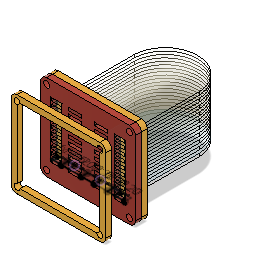
number_base_space_50mm_3mm_2mm v16 (Autodesk Fusion 360 design; units mm, degrees)
Autodesk Fusion 360 part; units mm, degrees
note: some values were not read from the file. Set by a fixed rule: which face or edge a step refers to.
(part 1 of 2)
sketch "Skizze1" plane through (0, 0, 0) normal (0, 1, 0) x (1, 0, 0)
  line L0 (0, 0) -> (43.75, 0)
  line L1 (43.75, 0) -> (43.75, -70)
  line L2 (43.75, -70) -> (0, -70)
  line L3 (0, -70) -> (0, 0)
  line L4 (36.1216, -93.0117) -> (36.1102, -92.9933) construction
  arc A0 (43.75, -23.3333) -> (0, -23.3333) centre (21.875, -21.9206) ccw
  line L5 (0, -70) -> (4, -70)
  line L6 (4, -70) -> (4, -74)
  line L7 (4, -74) -> (0, -74)
  line L8 (0, -74) -> (0, -70)
  line L9 (39.75, -70) -> (43.75, -70)
  line L10 (43.75, -70) -> (43.75, -74)
  line L11 (43.75, -74) -> (39.75, -74)
  line L12 (39.75, -74) -> (39.75, -70)
  line L13 (8.75, -70) -> (17.5, -70)
  line L14 (17.5, -70) -> (17.5, -74)
  line L15 (17.5, -74) -> (8.75, -74)
  line L16 (8.75, -74) -> (8.75, -70)
  line L17 (26.25, -70) -> (35, -70)
  line L18 (35, -70) -> (35, -74)
  line L19 (35, -74) -> (26.25, -74)
  line L20 (26.25, -74) -> (26.25, -70)
  line L21 (4, -70) -> (2.5, -70)
  line L22 (2.5029, -74) -> (4, -74)
  line L23 (4, -74) -> (4, -70)
  line L24 (39.75, -70) -> (41.25, -70)
  line L25 (39.75, -55) -> (39.75, -70)
  line L26 (43.75, -74) -> (46.75, -74)
  line L27 (46.75, -74) -> (46.75, -70)
  line L28 (46.75, -70) -> (43.75, -70)
  line L29 (43.75, -70) -> (43.75, -74)
  line L30 (0, -70) -> (-3, -70)
  line L31 (-3, -70) -> (-3, -74)
  line L32 (-3, -74) -> (0, -74)
  line L33 (0, -74) -> (0, -70)
  line L34 (-3, -70) -> (34.25, -70)
  line L35 (-3, -69.5) -> (-3, -70)
  line L36 (4, -70) -> (26.25, -70)
  line L37 (26.25, -70) -> (26.25, -74)
  line L38 (4, -74) -> (4, -70)
  line L39 (39.75, -70) -> (17.5, -70)
  line L40 (17.5, -70) -> (17.5, -74)
  line L41 (39.75, -74) -> (39.75, -70)
  point P0 (21.875, -70)
  dimension "d1" = 43.75
  dimension "d2" = 70
  dimension "d15" = 23.3333
  dimension "d16" = 23.3333
  dimension "d21" = 4
  dimension "d22" = 4
  dimension "d23" = 4
  dimension "d24" = 4
  dimension "d25" = 8.75
  dimension "d26" = 4
  dimension "d27" = 8.75
  dimension "d28" = 8.75
  dimension "d29" = 4
  dimension "d30" = 8.75
  dimension "d31" = 4
  dimension "d32" = 1.5
  dimension "d34" = 1.5
  dimension "d35" = 3
  dimension "d36" = 3
  dimension "d37" = 4
  dimension "d38" = 4
  dimension "d153" = 0.5
  constraint horizontal L0
  constraint vertical L1
  constraint horizontal L2
  constraint vertical L3
  constraint coincident L0.start L3.end
  constraint coincident L4 P0
  constraint midpoint L2 P0
  constraint coincident L3 A0.end
  constraint coincident L1 A0.start
  constraint tangent L0 A0
  constraint horizontal L5
  constraint vertical L6
  constraint horizontal L7
  constraint vertical L8
  constraint horizontal L9
  constraint vertical L10
  constraint horizontal L11
  constraint vertical L12
  constraint coincident L2 L9.start
  constraint coincident L1.end L10
  constraint horizontal L13
  constraint vertical L14
  constraint horizontal L15
  constraint vertical L16
  constraint coincident L2 L13.start
  constraint horizontal L17
  constraint vertical L18
  constraint horizontal L19
  constraint vertical L20
  constraint coincident L2 L17.start
  constraint horizontal L21
  constraint horizontal L22
  constraint vertical L23
  constraint horizontal L24
  constraint vertical L25
  constraint horizontal L26
  constraint vertical L27
  constraint horizontal L28
  constraint vertical L29
  constraint horizontal L30
  constraint vertical L31
  constraint horizontal L32
  constraint vertical L33
  constraint horizontal L34
  constraint vertical L35
  constraint horizontal L36
  constraint vertical L37
  constraint vertical L38
  constraint horizontal L39
  constraint vertical L40
  constraint vertical L41
  measures "d1" distance of L0.start L0.end
  measures "d2" distance of L0.start L2.end
  measures "d15" distance of L0.start A0.end
  measures "d16" distance of L0.end A0.start
  measures "d21" distance of L6.end L7.end
  measures "d22" distance of L10.end L11.end
  measures "d23" distance of L9.start L11.end
  measures "d24" distance of L5.end L6.end
  measures "d25" distance of L13.start L13.end
  measures "d26" distance of L13.start L15.end
  measures "d27" distance of L8 L16
  measures "d28" distance of L17.start L17.end
  measures "d29" distance of L17.start L19.end
  measures "d30" distance of L10 L18
  measures "d31" distance of L21.end L22.start
  measures "d32" distance of L5.end L21.end
  measures "d34" distance of L9.start L24.end
  measures "d35" distance of L10.end L26.end
  measures "d36" distance of L2.end L30.end
  measures "d37" distance of L26.end L27.end
  measures "d38" distance of L30.end L31.end
  measures "d153" distance of L30.end L35.start
extrude "Extrusion1" add sketch "Skizze1" along normal blind 2 contours L1 L2 L3 A0 L5 L9 L13 L17 L21 L24 L34 L36 L39 | L2 L5 L6 L7 L8 L21 L22 L23 L33 L34 L38 | L8 L30 L31 L32 L33 L34 | L2 L9 L10 L11 L12 L24 L29 L41 | L10 L26 L27 L28 L29 | L2 L13 L14 L15 L16 L34 L36 L40 | L2 L17 L18 L19 L20 L34 L37 L39 makes body 1
sketch "Skizze2" plane through (0, 0, 70) normal (0, 0, -1) x (-1, 0, 0)
  line L0 (0, 0) -> (3, 0)
  line L1 (3, 0) -> (3, 2)
  line L2 (3, 2) -> (0, 2)
  line L3 (0, 2) -> (0, 0)
  line L4 (0.1, -0.01) -> (-43.85, -0.01)
  line L5 (-43.85, -0.01) -> (-43.85, 38.01)
  line L6 (-43.85, 38.01) -> (0.1, 38.01)
  line L7 (0.1, 38.01) -> (0.1, -0.01)
  line L8 (0, 0) -> (-43.75, 0)
  line L9 (-43.75, 0) -> (-43.75, 2)
  line L10 (10.1, -10.01) -> (-53.85, -10.01)
  line L11 (-53.85, -10.01) -> (-53.85, 48.01)
  line L12 (-53.85, 48.01) -> (10.1, 48.01)
  line L13 (10.1, 48.01) -> (10.1, -10.01)
  circle A0 centre (-49.85, -6.01) radius 4
  circle A1 centre (6.1, 44.01) radius 4
  circle A2 centre (-49.85, 44.01) radius 4
  circle A3 centre (6.1, -6.01) radius 4
  circle A4 centre (6.1, -6.01) radius 2
  circle A5 centre (-49.85, -6.01) radius 2
  circle A6 centre (-49.85, 44.01) radius 2
  circle A7 centre (6.1, 44.01) radius 2
  line L14 (-80, 31) -> (-59, 31)
  line L15 (-59, 31) -> (-59, 29)
  line L16 (-59, 29) -> (-80, 29)
  line L17 (-80, 29) -> (-80, 31)
  line L18 (-100.8189, 25.8246) -> (-75.8188, 25.8008) construction
  line L19 (-75.8188, 25.8008) -> (-75.8107, 34.2225) construction
  line L20 (-75.8107, 34.2225) -> (-100.8108, 34.2463) construction
  line L21 (-100.8108, 34.2463) -> (-100.8189, 25.8246) construction
  line L22 (-81, 19) -> (-60, 19)
  line L23 (-60, 19) -> (-60, 15)
  line L24 (-60, 15) -> (-81, 15)
  line L25 (-81, 15) -> (-81, 19)
  line L26 (-106, 13) -> (-86, 13) construction
  line L27 (-86, 13) -> (-86, 18) construction
  line L28 (-86, 18) -> (-106, 18) construction
  line L29 (-106, 18) -> (-106, 13) construction
  dimension "d41" = 0.01
  dimension "d42" = 38.02
  dimension "d43" = 0.1
  dimension "d44" = 0.1
  dimension "d45" = 10
  dimension "d46" = 10
  dimension "d47" = 10
  dimension "d48" = 10
  dimension "d49" = 8
  dimension "d50" = 8
  dimension "d51" = 8
  dimension "d52" = 8
  dimension "d53" = 4
  dimension "d54" = 4
  dimension "d55" = 4
  dimension "d56" = 4
  dimension "d126" = 2
  dimension "d127" = 21
  dimension "d128" = 2
  dimension "d129" = 21
  dimension "d130" = 4
  dimension "d131" = 2
  constraint horizontal L4
  constraint vertical L5
  constraint horizontal L6
  constraint vertical L7
  constraint horizontal L10
  constraint vertical L11
  constraint horizontal L12
  constraint vertical L13
  constraint tangent L10 A0
  constraint tangent L11 A0
  constraint tangent L11 A2
  constraint tangent L12 A2
  constraint tangent L13 A3
  constraint tangent L10 A3
  constraint tangent L12 A1
  constraint tangent L13 A1
  constraint concentric A3 A4
  constraint concentric A0 A5
  constraint concentric A2 A6
  constraint concentric A1 A7
  constraint horizontal L14
  constraint vertical L15
  constraint horizontal L16
  constraint vertical L17
  constraint horizontal L22
  constraint vertical L23
  constraint horizontal L24
  constraint vertical L25
  measures "d41" distance of L4 L8
  measures "d42" distance of L4.start L6.end
  measures "d43" distance of L3 L7
  measures "d44" distance of L5 L9
  measures "d45" distance of L7 L13
  measures "d46" distance of L5 L11
  measures "d47" distance of L4 L10
  measures "d48" distance of L6 L12
  measures "d49" diameter of A3
  measures "d50" diameter of A0
  measures "d51" diameter of A2
  measures "d52" diameter of A1
  measures "d53" diameter of A4
  measures "d54" diameter of A5
  measures "d55" diameter of A6
  measures "d56" diameter of A7
  measures "d126" distance of L14.start L16.end
  measures "d127" distance of L14.start L14.end
  measures "d129" distance of L22.start L22.end
  measures "d130" distance of L22.start L24.end
extrude "Extrusion2" add sketch "Skizze2" along normal blind 4 separate body contours L0 L1 L2 L7 | L10 L11 L12 L13 A0 A1 A2 A3 | A3 | A0 | A1 | A2 makes body 2
copy_body "Körper kopieren/einfügen1" bodies 2 makes body 3
move_body "Verschieben1" bodies 3 to x (1, 0, 0) y (0, 1, 0) z (0, 0, 1) at (0, 0, 4)
extrude "Extrusion3" cut 3 faces at (-0.1, 1.3333, 72.6667) (-0.1, -0.0033, 72.6667) (-0.1, 26.0067, 71.3333) along direction (-1, 0, 0) blind 3.5 on bodies 3 bodies 3
extrude "Extrusion4" cut 1 faces at (43.85, 12.6633, 71.3333) along direction (1, 0, 0) blind 3.5 on bodies 3 bodies 3
sketch "Skizze3" plane through (0, 2, 0) normal (0, 1, 0) x (-1, 0, 0)
  line L0 (0, 70) -> (3, 70)
  line L1 (3, 70) -> (3, 74)
  line L2 (3, 74) -> (-4, 74)
  line L3 (-4, 74) -> (-4, 70)
  line L4 (-4, 70) -> (-8.75, 70)
  line L5 (-8.75, 70) -> (-8.75, 74)
  line L6 (-8.75, 74) -> (-17.5, 74)
  line L7 (-17.5, 74) -> (-17.5, 70)
  line L8 (-17.5, 70) -> (-26.25, 70)
  line L9 (-26.25, 70) -> (-26.25, 74)
  line L10 (-26.25, 74) -> (-35, 74)
  line L11 (-35, 74) -> (-35, 70)
  line L12 (-39.75, 70) -> (-39.75, 74)
  line L13 (-39.75, 74) -> (-46.75, 74)
  line L14 (-46.75, 74) -> (-46.75, 70)
  line L15 (-46.75, 70) -> (-43.75, 70)
  line L16 (-43.75, 70) -> (-43.75, 20.5078)
  arc A0 (-43.75, 20.5078) -> (0, 20.5078) centre (-21.875, 21.9206) ccw
  line L17 (0, 20.5078) -> (0, 70)
  line L18 (3, 70) -> (-4, 70)
  line L19 (-4, 70) -> (-4, 74)
  line L20 (-4, 74) -> (3, 74)
  line L21 (3, 74) -> (3, 70)
  line L22 (-8.75, 70) -> (-17.5, 70)
  line L23 (-17.5, 70) -> (-17.5, 74)
  line L24 (-17.5, 74) -> (-8.75, 74)
  line L25 (-8.75, 74) -> (-8.75, 70)
  line L26 (-26.25, 70) -> (-35, 70)
  line L27 (-35, 70) -> (-35, 74)
  line L28 (-35, 74) -> (-26.25, 74)
  line L29 (-26.25, 74) -> (-26.25, 70)
  line L30 (-39.75, 70) -> (-46.75, 70)
  line L31 (-46.75, 70) -> (-46.75, 74)
  line L32 (-46.75, 74) -> (-39.75, 74)
  line L33 (-39.75, 74) -> (-39.75, 70)
  line L34 (-17.5, 70) -> (-26.25, 70)
  line L35 (-26.25, 70) -> (-26.25, 74)
  line L36 (-26.25, 74) -> (-17.5, 74)
  line L37 (-17.5, 74) -> (-17.5, 70)
  line L38 (-35, 70) -> (-39.75, 70)
  line L39 (-39.75, 70) -> (-39.75, 74)
  line L40 (-39.75, 74) -> (-35, 74)
  line L41 (-35, 74) -> (-35, 70)
  line L42 (-4, 70) -> (-8.75, 70)
  line L43 (-8.75, 70) -> (-8.75, 74)
  line L44 (-8.75, 74) -> (-4, 74)
  line L45 (-4, 74) -> (-4, 70)
  line L46 (-4.2, 70) -> (-8.55, 70)
  line L47 (-8.55, 70) -> (-8.55, 74)
  line L48 (-8.55, 74) -> (-4.2, 74)
  line L49 (-4.2, 74) -> (-4.2, 70)
  line L50 (-17.7, 70) -> (-26.05, 70)
  line L51 (-26.05, 70) -> (-26.05, 74)
  line L52 (-26.05, 74) -> (-17.7, 74)
  line L53 (-17.7, 74) -> (-17.7, 70)
  line L54 (-35.2, 70) -> (-39.55, 70)
  line L55 (-39.55, 70) -> (-39.55, 74)
  line L56 (-39.55, 74) -> (-35.2, 74)
  line L57 (-35.2, 74) -> (-35.2, 70)
  line L58 (-35, 70) -> (-39.75, 70)
  dimension "d63" = 0.2
  dimension "d64" = 0.2
  dimension "d65" = 0.2
  dimension "d66" = 0.2
  dimension "d67" = 0.2
  dimension "d68" = 0.2
  constraint horizontal L18
  constraint vertical L19
  constraint horizontal L20
  constraint vertical L21
  constraint coincident L2.end L3.start
  constraint coincident L0.end L1.start
  constraint horizontal L22
  constraint vertical L23
  constraint horizontal L24
  constraint vertical L25
  constraint coincident L6.end L7.start
  constraint coincident L4.end L5.start
  constraint horizontal L26
  constraint vertical L27
  constraint horizontal L28
  constraint vertical L29
  constraint coincident L10.end L11.start
  constraint coincident L8.end L9.start
  constraint horizontal L30
  constraint vertical L31
  constraint horizontal L32
  constraint vertical L33
  constraint coincident L13.end L14.start
  constraint coincident L12.start L30.start
  constraint horizontal L34
  constraint vertical L35
  constraint horizontal L36
  constraint vertical L37
  constraint coincident L9.end L10.start
  constraint coincident L7.end L8.start
  constraint horizontal L38
  constraint vertical L39
  constraint horizontal L40
  constraint vertical L41
  constraint coincident L11.end L26.end
  constraint horizontal L42
  constraint vertical L43
  constraint horizontal L44
  constraint vertical L45
  constraint coincident L3.end L4.start
  constraint horizontal L46
  constraint vertical L47
  constraint horizontal L48
  constraint vertical L49
  constraint horizontal L50
  constraint vertical L51
  constraint horizontal L52
  constraint vertical L53
  constraint coincident L4.end L46
  constraint coincident L5.end L48
  constraint coincident L9.end L52
  constraint coincident L8.end L50
  constraint horizontal L54
  constraint vertical L55
  constraint horizontal L56
  constraint vertical L57
  constraint coincident L12.end L56
  constraint coincident L12.start L54
  measures "d63" distance of L33 L55
  measures "d64" distance of L27 L57
  measures "d65" distance of L29 L51
  measures "d66" distance of L37 L53
  measures "d67" distance of L43 L47
  measures "d68" distance of L45 L49
extrude "Extrusion5" add sketch "Skizze3" along normal blind 38.02 and the other way blind 4.5 contours L4 L42 L44 L46 L47 L48 L49 | L38 L40 L54 L55 L56 L57 L58 | L8 L34 L36 L50 L51 L52 L53 bodies 3
copy_body "Körper kopieren/einfügen2" bodies 3 makes body 4
move_body "Verschieben2" bodies 4 to x (1, 0, 0) y (0, 1, 0) z (0, 0, 1) at (0, 0, 22)
sketch "Skizze4" plane through (0, 0, 96) normal (0, 0, 1) x (1, 0, 0)
  line L0 (35.2, -0.01) -> (26.05, -0.01)
  line L1 (35.2, 38.01) -> (35.2, -0.01)
  line L2 (8.55, -0.01) -> (8.55, 38.01)
  line L3 (4.2, -0.01) -> (-3.6, -0.01)
  line L4 (-3.6, -0.01) -> (-3.6, 38.01)
  line L5 (4.2, 38.01) -> (4.2, -0.01)
  line L6 (39.55, -0.01) -> (39.55, 38.01)
  line L7 (26.05, 38.01) -> (35.2, 38.01)
  line L8 (47.35, 38.01) -> (47.35, -0.01)
  line L9 (47.35, -0.01) -> (39.55, -0.01)
  circle A0 centre (49.85, -6.01) radius 2
  circle A1 centre (49.85, 44.01) radius 2
  circle A2 centre (-6.1, 44.01) radius 2
  circle A3 centre (-6.1, -6.01) radius 2
  arc A4 (53.85, 44.01) -> (49.85, 48.01) centre (49.85, 44.01) ccw
  line L10 (49.85, 48.01) -> (-6.1, 48.01)
  arc A5 (-6.1, 48.01) -> (-10.1, 44.01) centre (-6.1, 44.01) ccw
  line L11 (-10.1, 44.01) -> (-10.1, -6.01)
  arc A6 (-10.1, -6.01) -> (-6.1, -10.01) centre (-6.1, -6.01) ccw
  line L12 (-6.1, -10.01) -> (49.85, -10.01)
  arc A7 (49.85, -10.01) -> (53.85, -6.01) centre (49.85, -6.01) ccw
  line L13 (53.85, -6.01) -> (53.85, 44.01)
  line L14 (-3.6, 38.01) -> (35.2, 38.01)
  line L15 (35.2, 38.01) -> (35.2, -0.01)
  line L16 (35.2, -0.01) -> (-3.6, -0.01)
  line L17 (-3.6, -0.01) -> (-3.6, 38.01)
  line L18 (-3.6, 38.01) -> (4.2, 38.01)
  line L19 (26.05, -0.01) -> (26.05, 38.01)
  line L20 (17.7, -0.01) -> (8.55, -0.01)
  line L21 (8.55, 38.01) -> (17.7, 38.01)
  line L22 (17.7, 38.01) -> (17.7, -0.01)
  line L23 (39.55, 38.01) -> (47.35, 38.01)
  constraint horizontal L14
  constraint vertical L15
  constraint horizontal L16
  constraint vertical L17
  constraint coincident L4.end L17
  constraint coincident L3.end L16
  constraint coincident L1.start L15
  constraint coincident L1.start L14
extrude "Extrusion6" add sketch "Skizze4" against normal blind 2 contours L0 L1 L7 L14 L15 L16 L19 | L2 L14 L16 L20 L21 L22 | L3 L4 L5 L14 L16 L17 L18 bodies 4
move_body "Verschieben3" bodies 4 to x (1, 0, 0) y (0, 1, 0) z (0, 0, 1) at (0, 0, 7)
copy_body "Körper kopieren/einfügen3" bodies 4 makes body 5
move_body "Verschieben4" bodies 5 to x (1, 0, 0) y (0, 1, 0) z (0, 0, 1) at (0, 0, -9)
sketch "Skizze5" plane through (0, 0, 94) normal (0, 0, 1) x (1, 0, 0)
  circle A0 centre (49.85, -6.01) radius 2
  circle A1 centre (49.85, 44.01) radius 2
  circle A2 centre (-6.1, 44.01) radius 2
  circle A3 centre (-6.1, -6.01) radius 2
  arc A4 (53.85, 44.01) -> (49.85, 48.01) centre (49.85, 44.01) ccw
  line L0 (49.85, 48.01) -> (-6.1, 48.01)
  arc A5 (-6.1, 48.01) -> (-10.1, 44.01) centre (-6.1, 44.01) ccw
  line L1 (-10.1, 44.01) -> (-10.1, -6.01)
  arc A6 (-10.1, -6.01) -> (-6.1, -10.01) centre (-6.1, -6.01) ccw
  line L2 (-6.1, -10.01) -> (49.85, -10.01)
  arc A7 (49.85, -10.01) -> (53.85, -6.01) centre (49.85, -6.01) ccw
  line L3 (53.85, -6.01) -> (53.85, 44.01)
  line L4 (-6.1, 44.01) -> (49.85, 44.01)
  line L5 (49.85, 44.01) -> (49.85, -6.01)
  line L6 (49.85, -6.01) -> (-6.1, -6.01)
  line L7 (-6.1, -6.01) -> (-6.1, 44.01)
  line L8 (39.55, -0.01) -> (39.55, 38.01)
  line L9 (39.55, 38.01) -> (47.35, 38.01)
  line L10 (47.35, 38.01) -> (47.35, -0.01)
  line L11 (47.35, -0.01) -> (39.55, -0.01)
  constraint horizontal L4
  constraint vertical L5
  constraint horizontal L6
  constraint vertical L7
  constraint coincident A2.centre L7
  constraint coincident A2.centre L4
  constraint coincident A0.centre L6
  constraint coincident A0.centre L5
extrude "Extrusion7" cut sketch "Skizze5" against normal blind 4 contours A0 A1 A2 A3 L4 L5 L6 L7 | L8 L9 L10 L11 bodies 5
copy_body "Körper kopieren/einfügen4" bodies 3 makes body 6
move_body "Verschieben5" bodies 6 to x (1, 0, 0) y (0, 1, 0) z (0, 0, 1) at (0, 0, 4)
sketch "Skizze6" plane through (0, 0, 78) normal (0, 0, 1) x (1, 0, 0)
  line L0 (35.2, -0.01) -> (26.05, -0.01)
  line L1 (35.2, 38.01) -> (35.2, -0.01)
  line L2 (4.2, -0.01) -> (-3.6, -0.01)
  line L3 (-3.6, -0.01) -> (-3.6, 38.01)
  line L4 (4.2, 38.01) -> (4.2, -0.01)
  circle A0 centre (49.85, 44.01) radius 2
  circle A1 centre (49.85, -6.01) radius 2
  circle A2 centre (-6.1, -6.01) radius 2
  circle A3 centre (-6.1, 44.01) radius 2
  arc A4 (53.85, 44.01) -> (49.85, 48.01) centre (49.85, 44.01) ccw
  line L5 (49.85, 48.01) -> (-6.1, 48.01)
  arc A5 (-6.1, 48.01) -> (-10.1, 44.01) centre (-6.1, 44.01) ccw
  line L6 (-10.1, 44.01) -> (-10.1, -6.01)
  arc A6 (-10.1, -6.01) -> (-6.1, -10.01) centre (-6.1, -6.01) ccw
  line L7 (-6.1, -10.01) -> (49.85, -10.01)
  arc A7 (49.85, -10.01) -> (53.85, -6.01) centre (49.85, -6.01) ccw
  line L8 (53.85, -6.01) -> (53.85, 44.01)
  line L9 (39.55, -0.01) -> (39.55, 38.01)
  line L10 (26.05, 38.01) -> (35.2, 38.01)
  line L11 (47.35, 38.01) -> (47.35, -0.01)
  line L12 (47.35, -0.01) -> (39.55, -0.01)
  line L13 (8.55, -0.01) -> (8.55, 38.01)
  line L14 (26.05, 38.01) -> (47.35, 38.01)
  line L15 (47.35, 38.01) -> (47.35, -0.01)
  line L16 (47.35, -0.01) -> (26.05, -0.01)
  line L17 (26.05, -0.01) -> (26.05, 38.01)
  line L18 (47.35, -0.01) -> (26.05, -0.01)
  line L19 (26.05, -0.01) -> (26.05, 38.01)
  line L20 (26.05, 38.01) -> (47.35, 38.01)
  line L21 (47.35, 38.01) -> (47.35, -0.01)
  line L22 (4.2, -0.01) -> (-3.6, -0.01)
  line L23 (-3.6, -0.01) -> (-3.6, 38.01)
  line L24 (-3.6, 38.01) -> (4.2, 38.01)
  line L25 (4.2, 38.01) -> (4.2, -0.01)
  line L26 (35.2, 0) -> (26.05, 0)
  line L27 (26.05, 0) -> (26.05, 2)
  line L28 (26.05, 2) -> (35.2, 2)
  line L29 (35.2, 2) -> (35.2, 0)
  line L30 (17.7, -0.01) -> (8.55, -0.01)
  line L31 (8.55, -0.01) -> (8.55, 0)
  line L32 (8.55, 0) -> (17.7, 0)
  line L33 (17.7, 0) -> (17.7, -0.01)
  line L34 (17.7, 0) -> (8.55, 0)
  line L35 (8.55, 0) -> (8.55, 2)
  line L36 (8.55, 2) -> (17.7, 2)
  line L37 (17.7, 2) -> (17.7, 0)
  line L38 (17.7, 2) -> (8.55, 2)
  line L39 (8.55, 2) -> (8.55, 4)
  line L40 (8.55, 4) -> (17.7, 4)
  line L41 (17.7, 4) -> (17.7, 2)
  line L42 (17.7, 4) -> (8.55, 4)
  line L43 (8.55, 4) -> (8.55, 6)
  line L44 (8.55, 6) -> (17.7, 6)
  line L45 (17.7, 6) -> (17.7, 4)
  line L46 (26.05, 0) -> (35.2, 0)
  line L47 (35.2, 0) -> (35.2, -0.01)
  line L48 (35.2, -0.01) -> (26.05, -0.01)
  line L49 (26.05, -0.01) -> (26.05, 0)
  line L50 (8.55, 8) -> (17.7, 8)
  line L51 (17.7, 8) -> (17.7, 6)
  line L52 (17.7, 6) -> (8.55, 6)
  line L53 (8.55, 6) -> (8.55, 8)
  line L54 (8.55, 10) -> (17.7, 10)
  line L55 (17.7, 10) -> (17.7, 8)
  line L56 (17.7, 8) -> (8.55, 8)
  line L57 (8.55, 8) -> (8.55, 10)
  line L58 (8.55, 12) -> (17.7, 12)
  line L59 (17.7, 12) -> (17.7, 10)
  line L60 (17.7, 10) -> (8.55, 10)
  line L61 (8.55, 10) -> (8.55, 12)
  line L62 (8.55, 14) -> (17.7, 14)
  line L63 (17.7, 14) -> (17.7, 12)
  line L64 (17.7, 12) -> (8.55, 12)
  line L65 (8.55, 12) -> (8.55, 14)
  line L66 (8.55, 16) -> (17.7, 16)
  line L67 (17.7, 16) -> (17.7, 14)
  line L68 (17.7, 14) -> (8.55, 14)
  line L69 (8.55, 14) -> (8.55, 16)
  line L70 (8.55, 18) -> (17.7, 18)
  line L71 (17.7, 18) -> (17.7, 16)
  line L72 (17.7, 16) -> (8.55, 16)
  line L73 (8.55, 16) -> (8.55, 18)
  line L74 (8.55, 20) -> (17.7, 20)
  line L75 (17.7, 20) -> (17.7, 18)
  line L76 (17.7, 18) -> (8.55, 18)
  line L77 (8.55, 18) -> (8.55, 20)
  line L78 (26.05, 20) -> (35.2, 20)
  line L79 (35.2, 20) -> (35.2, 18)
  line L80 (35.2, 18) -> (26.05, 18)
  line L81 (26.05, 18) -> (26.05, 20)
  line L82 (26.05, 18) -> (35.2, 18)
  line L83 (35.2, 18) -> (35.2, 16)
  line L84 (35.2, 16) -> (26.05, 16)
  line L85 (26.05, 16) -> (26.05, 18)
  line L86 (26.05, 16) -> (35.2, 16)
  line L87 (35.2, 16) -> (35.2, 14)
  line L88 (35.2, 14) -> (26.05, 14)
  line L89 (26.05, 14) -> (26.05, 16)
  line L90 (26.05, 14) -> (35.2, 14)
  line L91 (35.2, 14) -> (35.2, 12)
  line L92 (35.2, 12) -> (26.05, 12)
  line L93 (26.05, 12) -> (26.05, 14)
  line L94 (26.05, 12) -> (35.2, 12)
  line L95 (35.2, 12) -> (35.2, 10)
  line L96 (35.2, 10) -> (26.05, 10)
  line L97 (26.05, 10) -> (26.05, 12)
  line L98 (26.05, 10) -> (35.2, 10)
  line L99 (35.2, 10) -> (35.2, 8)
  line L100 (35.2, 8) -> (26.05, 8)
  line L101 (26.05, 8) -> (26.05, 10)
  line L102 (26.05, 8) -> (35.2, 8)
  line L103 (35.2, 8) -> (35.2, 6)
  line L104 (35.2, 6) -> (26.05, 6)
  line L105 (26.05, 6) -> (26.05, 8)
  line L106 (26.05, 6) -> (35.2, 6)
  line L107 (35.2, 6) -> (35.2, 4)
  line L108 (35.2, 4) -> (26.05, 4)
  line L109 (26.05, 4) -> (26.05, 6)
  line L110 (26.05, 4) -> (35.2, 4)
  line L111 (35.2, 4) -> (35.2, 2)
  line L112 (35.2, 2) -> (26.05, 2)
  line L113 (26.05, 2) -> (26.05, 4)
  line L114 (8.55, 38.01) -> (17.7, 38.01)
  line L115 (17.7, 38.01) -> (17.7, 38)
  line L116 (17.7, 38) -> (8.55, 38)
  line L117 (8.55, 38) -> (8.55, 38.01)
  line L118 (27.8, 38.01) -> (35.2, 38.01)
  line L119 (35.2, 38.01) -> (35.2, 38)
  line L120 (35.2, 38) -> (27.8, 38)
  line L121 (27.8, 38) -> (27.8, 38.01)
  line L122 (-3.6, 38.01) -> (4.2, 38.01)
  line L123 (8.55, 22) -> (17.7, 22)
  line L124 (17.7, 22) -> (17.7, 20)
  line L125 (17.7, 20) -> (8.55, 20)
  line L126 (8.55, 20) -> (8.55, 22)
  line L127 (8.55, 24) -> (17.7, 24)
  line L128 (17.7, 24) -> (17.7, 22)
  line L129 (17.7, 22) -> (8.55, 22)
  line L130 (8.55, 22) -> (8.55, 24)
  line L131 (8.55, 26) -> (17.7, 26)
  line L132 (17.7, 26) -> (17.7, 24)
  line L133 (17.7, 24) -> (8.55, 24)
  line L134 (8.55, 24) -> (8.55, 26)
  line L135 (26.05, 26) -> (35.2, 26)
  line L136 (35.2, 26) -> (35.2, 24)
  line L137 (35.2, 24) -> (26.05, 24)
  line L138 (26.05, 24) -> (26.05, 26)
  line L139 (26.05, 24) -> (35.2, 24)
  line L140 (35.2, 24) -> (35.2, 22)
  line L141 (35.2, 22) -> (26.05, 22)
  line L142 (26.05, 22) -> (26.05, 24)
  line L143 (26.05, 22) -> (35.2, 22)
  line L144 (35.2, 22) -> (35.2, 20)
  line L145 (35.2, 20) -> (26.05, 20)
  line L146 (26.05, 20) -> (26.05, 22)
  line L147 (8.55, 28) -> (17.7, 28)
  line L148 (17.7, 28) -> (17.7, 26)
  line L149 (17.7, 26) -> (8.55, 26)
  line L150 (8.55, 26) -> (8.55, 28)
  line L151 (26.05, 28) -> (35.2, 28)
  line L152 (35.2, 28) -> (35.2, 26)
  line L153 (35.2, 26) -> (26.05, 26)
  line L154 (26.05, 26) -> (26.05, 28)
  line L155 (8.55, 38) -> (17.7, 38)
  line L156 (17.7, 38) -> (17.7, 36)
  line L157 (17.7, 36) -> (8.55, 36)
  line L158 (8.55, 36) -> (8.55, 38)
  line L159 (8.55, 36) -> (17.7, 36)
  line L160 (17.7, 36) -> (17.7, 34)
  line L161 (17.7, 34) -> (8.55, 34)
  line L162 (8.55, 34) -> (8.55, 36)
  line L163 (8.55, 34) -> (17.7, 34)
  line L164 (17.7, 34) -> (17.7, 32)
  line L165 (17.7, 32) -> (8.55, 32)
  line L166 (8.55, 32) -> (8.55, 34)
  line L167 (8.55, 32) -> (17.7, 32)
  line L168 (17.7, 32) -> (17.7, 30)
  line L169 (17.7, 30) -> (8.55, 30)
  line L170 (8.55, 30) -> (8.55, 32)
  line L171 (8.55, 30) -> (17.7, 30)
  line L172 (17.7, 30) -> (17.7, 28)
  line L173 (17.7, 28) -> (8.55, 28)
  line L174 (8.55, 28) -> (8.55, 30)
  line L175 (26.05, 38) -> (35.2, 38)
  line L176 (35.2, 38) -> (35.2, 36)
  line L177 (35.2, 36) -> (26.05, 36)
  line L178 (26.05, 36) -> (26.05, 38)
  line L179 (26.05, 36) -> (35.2, 36)
  line L180 (35.2, 36) -> (35.2, 34)
  line L181 (35.2, 34) -> (26.05, 34)
  line L182 (26.05, 34) -> (26.05, 36)
  line L183 (26.05, 34) -> (35.2, 34)
  line L184 (35.2, 34) -> (35.2, 32)
  line L185 (35.2, 32) -> (26.05, 32)
  line L186 (26.05, 32) -> (26.05, 34)
  line L187 (26.05, 32) -> (35.2, 32)
  line L188 (35.2, 32) -> (35.2, 30)
  line L189 (35.2, 30) -> (26.05, 30)
  line L190 (26.05, 30) -> (26.05, 32)
  line L191 (26.05, 30) -> (35.2, 30)
  line L192 (35.2, 30) -> (35.2, 28)
  line L193 (35.2, 28) -> (26.05, 28)
  line L194 (26.05, 28) -> (26.05, 30)
  line L195 (26.05, -0.01) -> (26.05, 38.01)
  line L196 (17.7, -0.01) -> (8.55, -0.01)
  line L197 (8.55, 38.01) -> (17.7, 38.01)
  line L198 (17.7, 38.01) -> (17.7, -0.01)
  line L199 (39.55, 38.01) -> (47.35, 38.01)
  dimension "d78" = 0.01
  dimension "d79" = 0.01
  dimension "d80" = 2
  dimension "d81" = 2
  dimension "d82" = 2
  dimension "d83" = 2
  dimension "d84" = 2
  dimension "d85" = 2
  dimension "d86" = 2
  dimension "d87" = 2
  dimension "d88" = 2
  dimension "d89" = 2
  dimension "d90" = 2
  dimension "d91" = 0.01
  dimension "d92" = 2
  dimension "d93" = 2
  dimension "d94" = 2
  dimension "d95" = 2
  dimension "d96" = 2
  dimension "d97" = 2
  dimension "d98" = 2
  dimension "d99" = 2
  dimension "d100" = 2
  dimension "d101" = 0.01
  dimension "d132" = 2
  dimension "d133" = 2
  dimension "d134" = 2
  dimension "d135" = 2
  dimension "d136" = 2
  dimension "d137" = 2
  dimension "d138" = 2
  dimension "d139" = 2
  dimension "d140" = 2
  dimension "d141" = 2
  dimension "d142" = 2
  dimension "d143" = 2
  dimension "d144" = 2
  dimension "d146" = 2
  dimension "d147" = 2
  dimension "d148" = 2
  dimension "d149" = 2
  dimension "d150" = 2
  constraint horizontal L14
  constraint vertical L15
  constraint horizontal L16
  constraint vertical L17
  constraint coincident L11.end L12.start
  constraint coincident L10.start L14.start
  constraint horizontal L18
  constraint vertical L19
  constraint horizontal L20
  constraint vertical L21
  constraint horizontal L22
  constraint vertical L23
  constraint horizontal L24
  constraint vertical L25
  constraint coincident L11.end L18
  constraint coincident L10.start L20
  constraint coincident L11.end L21
  constraint coincident L0.end L16.end
  constraint coincident L2.start L25
  constraint coincident L2.start L22
  constraint coincident L3.end L24
  constraint coincident L3.end L23
  constraint horizontal L26
  constraint vertical L27
  constraint horizontal L28
  constraint vertical L29
  constraint horizontal L30
  constraint vertical L31
  constraint horizontal L32
  constraint vertical L33
  constraint horizontal L34
  constraint vertical L35
  constraint horizontal L36
  constraint vertical L37
  constraint horizontal L38
  constraint vertical L39
  constraint horizontal L40
  constraint vertical L41
  constraint horizontal L42
  constraint vertical L43
  constraint horizontal L44
  constraint vertical L45
  constraint horizontal L46
  constraint vertical L47
  constraint horizontal L48
  constraint vertical L49
  constraint coincident L0.start L48
  constraint coincident L0.start L47
  constraint coincident L13.start L31
  constraint coincident L32.end L37
  constraint coincident L32.end L34
  constraint coincident L29 L26.start
  constraint coincident L26 L29.end
  constraint coincident L27 L26.end
  constraint coincident L31.end L35
  constraint coincident L36.end L41
  constraint coincident L36.end L38
  constraint coincident L40.end L45
  constraint coincident L40.end L42
  constraint coincident L35.end L39
  constraint coincident L39.end L43
  constraint horizontal L50
  constraint vertical L51
  constraint horizontal L52
  constraint vertical L53
  constraint horizontal L54
  constraint vertical L55
  constraint horizontal L56
  constraint vertical L57
  constraint horizontal L58
  constraint vertical L59
  constraint horizontal L60
  constraint vertical L61
  constraint horizontal L62
  constraint vertical L63
  constraint horizontal L64
  constraint vertical L65
  constraint horizontal L66
  constraint vertical L67
  constraint horizontal L68
  constraint vertical L69
  constraint horizontal L70
  constraint vertical L71
  constraint horizontal L72
  constraint vertical L73
  constraint horizontal L74
  constraint vertical L75
  constraint horizontal L76
  constraint vertical L77
  constraint horizontal L78
  constraint vertical L79
  constraint horizontal L80
  constraint vertical L81
  constraint horizontal L82
  constraint vertical L83
  constraint horizontal L84
  constraint vertical L85
  constraint horizontal L86
  constraint vertical L87
  constraint horizontal L88
  constraint vertical L89
  constraint horizontal L90
  constraint vertical L91
  constraint horizontal L92
  constraint vertical L93
  constraint horizontal L94
  constraint vertical L95
  constraint horizontal L96
  constraint vertical L97
  constraint horizontal L98
  constraint vertical L99
  constraint horizontal L100
  constraint vertical L101
  constraint horizontal L102
  constraint vertical L103
  constraint horizontal L104
  constraint vertical L105
  constraint horizontal L106
  constraint vertical L107
  constraint horizontal L108
  constraint vertical L109
  constraint horizontal L110
  constraint vertical L111
  constraint horizontal L112
  constraint vertical L113
  constraint coincident L44.end L51
  constraint coincident L44.end L52
  constraint coincident L43.end L53
  constraint coincident L50.end L55
  constraint coincident L50.end L56
  constraint coincident L54.end L59
  constraint coincident L54.end L60
  constraint coincident L58.end L63
  constraint coincident L58.end L64
  constraint coincident L62.end L67
  constraint coincident L62.end L68
  constraint coincident L66.end L71
  constraint coincident L66.end L72
  constraint coincident L70.end L75
  constraint coincident L70.end L76
  constraint coincident L50.start L57
  constraint coincident L54.start L61
  constraint coincident L58.start L65
  constraint coincident L62.start L69
  constraint coincident L66.start L73
  constraint coincident L70.start L77
  constraint horizontal L114
  constraint vertical L115
  constraint horizontal L116
  constraint vertical L117
  constraint horizontal L118
  constraint vertical L119
  constraint horizontal L120
  constraint vertical L121
  constraint coincident L13.end L117
  constraint coincident L13.end L114
  constraint coincident L74.end L115
  constraint coincident L28.end L111
  constraint coincident L28.end L112
  constraint coincident L107 L108.start
  constraint coincident L108 L107.end
  constraint coincident L103 L104.start
  constraint coincident L104 L103.end
  constraint coincident L99 L100.start
  constraint coincident L100 L99.end
  constraint coincident L95 L96.start
  constraint coincident L96 L95.end
  constraint coincident L91 L92.start
  constraint coincident L92 L91.end
  constraint coincident L87 L88.start
  constraint coincident L88 L87.end
  constraint coincident L83 L84.start
  constraint coincident L84 L83.end
  constraint coincident L79 L80.start
  constraint coincident L80 L79.end
  constraint coincident L27.end L113
  constraint coincident L109 L108.end
  constraint coincident L105 L104.end
  constraint coincident L101 L100.end
  constraint coincident L97 L96.end
  constraint coincident L93 L92.end
  constraint coincident L89 L88.end
  constraint coincident L85 L84.end
  constraint coincident L81 L80.end
  constraint coincident L1.start L119
  constraint horizontal L123
  constraint vertical L124
  constraint horizontal L125
  constraint vertical L126
  constraint horizontal L127
  constraint vertical L128
  constraint horizontal L129
  constraint vertical L130
  constraint horizontal L131
  constraint vertical L132
  constraint horizontal L133
  constraint vertical L134
  constraint horizontal L135
  constraint vertical L136
  constraint horizontal L137
  constraint vertical L138
  constraint horizontal L139
  constraint vertical L140
  constraint horizontal L141
  constraint vertical L142
  constraint horizontal L143
  constraint vertical L144
  constraint horizontal L145
  constraint vertical L146
  constraint horizontal L147
  constraint vertical L148
  constraint horizontal L149
  constraint vertical L150
  constraint horizontal L151
  constraint vertical L152
  constraint horizontal L153
  constraint vertical L154
  constraint coincident L74.end L124
  constraint coincident L74.end L125
  constraint coincident L123.end L128
  constraint coincident L123.end L129
  constraint coincident L127.end L132
  constraint coincident L127.end L133
  constraint coincident L131.end L148
  constraint coincident L131.end L149
  constraint coincident L78.end L144
  constraint coincident L78.end L145
  constraint coincident L140 L141.start
  constraint coincident L141 L140.end
  constraint coincident L136 L137.start
  constraint coincident L137 L136.end
  constraint coincident L135.end L152
  constraint coincident L135.end L153
  constraint coincident L78.start L146
  constraint coincident L142 L141.end
  constraint coincident L138 L137.end
  constraint coincident L135.start L154
  constraint coincident L74.start L126
  constraint coincident L123.start L130
  constraint coincident L127.start L134
  constraint coincident L131.start L150
  constraint horizontal L155
  constraint vertical L156
  constraint horizontal L157
  constraint vertical L158
  constraint horizontal L159
  constraint vertical L160
  constraint horizontal L161
  constraint vertical L162
  constraint horizontal L163
  constraint vertical L164
  constraint horizontal L165
  constraint vertical L166
  constraint horizontal L167
  constraint vertical L168
  constraint horizontal L169
  constraint vertical L170
  constraint horizontal L171
  constraint vertical L172
  constraint horizontal L173
  constraint vertical L174
  constraint horizontal L175
  constraint vertical L176
  constraint horizontal L177
  constraint vertical L178
  constraint horizontal L179
  constraint vertical L180
  constraint horizontal L181
  constraint vertical L182
  constraint horizontal L183
  constraint vertical L184
  constraint horizontal L185
  constraint vertical L186
  constraint horizontal L187
  constraint vertical L188
  constraint horizontal L189
  constraint vertical L190
  constraint horizontal L191
  constraint vertical L192
  constraint horizontal L193
  constraint vertical L194
  constraint coincident L147.end L172
  constraint coincident L147.end L173
  constraint coincident L168 L169.start
  constraint coincident L169 L168.end
  constraint coincident L147.start L174
  constraint coincident L170 L169.end
  constraint coincident L164 L165.start
  constraint coincident L165 L164.end
  constraint coincident L160 L161.start
  constraint coincident L161 L160.end
  constraint coincident L166 L165.end
  constraint coincident L162 L161.end
  constraint coincident L156 L157.start
  constraint coincident L157 L156.end
  constraint coincident L158 L157.end
  constraint coincident L151.end L192
  constraint coincident L151.end L193
  constraint coincident L188 L189.start
  constraint coincident L151.start L194
  constraint coincident L189 L188.end
  constraint coincident L190 L189.end
  constraint coincident L184 L185.start
  constraint coincident L185 L184.end
  constraint coincident L186 L185.end
  constraint coincident L180 L181.start
  constraint coincident L181 L180.end
  constraint coincident L182 L181.end
  constraint coincident L176 L177.start
  constraint coincident L177 L176.end
  constraint coincident L178 L177.end
  constraint coincident L156 L114.end
  measures "d78" distance of L26.end L0.end
  measures "d79" distance of L13.start L31.end
  measures "d80" distance of L31.end L35.end
  measures "d81" distance of L26.end L27.end
  measures "d82" distance of L35.end L39.end
  measures "d83" distance of L39.end L43.end
  measures "d84" distance of L50.start L43.end
  measures "d85" distance of L54.start L50.start
  measures "d86" distance of L58.start L54.start
  measures "d87" distance of L62.start L58.start
  measures "d88" distance of L66.start L62.start
  measures "d89" distance of L70.start L66.start
  measures "d90" distance of L74.start L70.start
  measures "d91" distance of L13.end L116.end
  measures "d92" distance of L108.end L27.end
  measures "d93" distance of L104.end L108.end
  measures "d94" distance of L100.end L104.end
  measures "d95" distance of L96.end L100.end
  measures "d96" distance of L92.end L96.end
  measures "d97" distance of L88.end L92.end
  measures "d98" distance of L84.end L88.end
  measures "d99" distance of L80.end L84.end
  measures "d100" distance of L78.start L80.end
  measures "d101" distance of L1.start L119.end
  measures "d132" distance of L123.start L74.start
  measures "d133" distance of L127.start L123.start
  measures "d134" distance of L131.start L127.start
  measures "d135" distance of L147.start L131.start
  measures "d136" distance of L141.end L78.start
  measures "d137" distance of L137.end L141.end
  measures "d138" distance of L135.start L137.end
  measures "d139" distance of L151.start L135.start
  measures "d140" distance of L169.end L147.start
  measures "d141" distance of L165.end L169.end
  measures "d142" distance of L161.end L165.end
  measures "d143" distance of L157.end L161.end
  measures "d144" distance of L116.end L157.end
  measures "d146" distance of L189.end L151.start
  measures "d147" distance of L185.end L189.end
  measures "d148" distance of L181.end L185.end
  measures "d149" distance of L177.end L181.end
  measures "d150" distance of L175.start L177.end
extrude "Extrusion20" add sketch "Skizze6" against normal blind 4 contours L0 L1 L16 L17 L18 L19 L26 L46 L47 L48 L49 L195 | L1 L17 L19 L26 L27 L28 L29 L46 L112 L195 | L1 L17 L19 L28 L108 L110 L111 L112 L113 L195 | L1 L10 L14 L20 L118 L119 L120 L121 L175 | L1 L17 L19 L100 L102 L103 L104 L105 L106 L195 | L1 L17 L19 L96 L98 L99 L100 L101 L102 L195 | L1 L17 L19 L177 L179 L180 L181 L182 L183 L195 | L1 L17 L19 L92 L94 L95 L96 L97 L98 L195 | L1 L17 L19 L181 L183 L184 L185 L186 L187 L195 | L1 L17 L19 L185 L187 L188 L189 L190 L191 L195 | L1 L17 L19 L84 L86 L87 L88 L89 L90 L195 | L1 L17 L19 L80 L82 L83 L84 L85 L86 L195 | L1 L17 L19 L135 L151 L152 L153 L154 L193 L195 | L1 L17 L19 L78 L79 L80 L81 L82 L145 L195 | L1 L17 L19 L135 L136 L137 L138 L139 L153 L195 | L1 L17 L19 L137 L139 L140 L141 L142 L143 L195 | L13 L30 L31 L32 L33 L34 L196 L198 | L13 L36 L38 L39 L40 L41 L42 L198 | L13 L40 L42 L43 L44 L45 L52 L198 | L13 L44 L50 L51 L52 L53 L56 L198 | L13 L54 L58 L59 L60 L61 L64 L198 | L13 L58 L62 L63 L64 L65 L68 L198 | L13 L62 L66 L67 L68 L69 L72 L198 | L13 L70 L74 L75 L76 L77 L125 L198 | L13 L74 L123 L124 L125 L126 L129 L198 | L13 L123 L127 L128 L129 L130 L133 L198 | L13 L131 L147 L148 L149 L150 L173 L198 | L13 L147 L169 L171 L172 L173 L174 L198 | L13 L165 L167 L168 L169 L170 L171 L198 | L13 L157 L159 L160 L161 L162 L163 L198 | L13 L116 L155 L156 L157 L158 L159 L198 | L13 L114 L115 L116 L117 L155 L197 L198 bodies 6
copy_body "Körper kopieren/einfügen14" bodies 6 makes body 7
move_body "Verschieben15" bodies 7 to x (1, 0, 0) y (0, 1, 0) z (0, 0, 1) at (0, 0, 4)
copy_body "Körper kopieren/einfügen15" bodies 1 makes body 8
move_body "Verschieben16" bodies 8 to x (1, 0, 0) y (0, 1, 0) z (0, 0, 1) at (0, 4, 0)
copy_body "Körper kopieren/einfügen16" bodies 8 makes body 9
move_body "Verschieben17" bodies 9 to x (1, 0, 0) y (0, 1, 0) z (0, 0, 1) at (0, 4, 0)
copy_body "Körper kopieren/einfügen17" bodies 9 makes body 10
move_body "Verschieben18" bodies 10 to x (1, 0, 0) y (0, 1, 0) z (0, 0, 1) at (0, 4, 0)
copy_body "Körper kopieren/einfügen18" bodies 10 makes body 11
move_body "Verschieben19" bodies 11 to x (1, 0, 0) y (0, 1, 0) z (0, 0, 1) at (0, 4, 0)
copy_body "Körper kopieren/einfügen19" bodies 11 makes body 12
move_body "Verschieben20" bodies 12 to x (1, 0, 0) y (0, 1, 0) z (0, 0, 1) at (0, 4, 0)
copy_body "Körper kopieren/einfügen20" bodies 12 makes body 13
move_body "Verschieben21" bodies 13 to x (1, 0, 0) y (0, 1, 0) z (0, 0, 1) at (0, 4, 0)
copy_body "Körper kopieren/einfügen21" bodies 13 makes body 14
move_body "Verschieben22" bodies 14 to x (1, 0, 0) y (0, 1, 0) z (0, 0, 1) at (0, 4, 0)
copy_body "Körper kopieren/einfügen22" bodies 14 makes body 15
move_body "Verschieben23" bodies 15 to x (1, 0, 0) y (0, 1, 0) z (0, 0, 1) at (0, 4, 0)
copy_body "Körper kopieren/einfügen24" bodies 15 makes body 16
move_body "Verschieben25" bodies 16 to x (1, 0, 0) y (0, 1, 0) z (0, 0, 1) at (0, 4, 0)
move_body "Verschieben26" bodies 3 to x (1, 0, 0) y (0, 1, 0) z (0, 0, 1) at (0, 0, 20)
move_body "Verschieben27" bodies 6 to x (1, 0, 0) y (0, 1, 0) z (0, 0, 1) at (0, 0, -4)